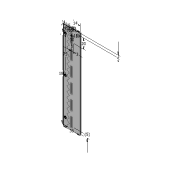
# Autodesk Inventor part: tray_side_top
Saved by Autodesk Inventor 2022 (Build 260153000, 153)
## iProperties
Created: 2022-05-19
Part Number: tray_side_top
Material: Generic
Document SubType Name: Modeling
Designer: Thomas
Density: 1 g/cm^3
Appearance: Default
Author: Thomas
Autodesk Inventor part; units mm, degrees
ref_plane "YZ Plane" through (0, 0, 0) normal (1, 0, 0) x (0, 1, 0)
ref_plane "XZ Plane" through (0, 0, 0) normal (0, 1, 0) x (-1, 0, 0)
ref_plane "XY Plane" through (0, 0, 0) normal (0, 0, 1) x (1, 0, 0)
sketch "Sketch1" plane through (0, 0, 0) normal (0, 0, 1) x (1, 0, 0)
  line L0 (0, 0) -> (-35, 0)
  line L1 (-35, 0) -> (-35, -180)
  line L2 (-35, -180) -> (0, -180)
  line L3 (0, -180) -> (0, 0)
  line L4 (-17, -5) -> (-14, -5)
  line L5 (-14, -5) -> (-14, -25)
  line L6 (-14, -25) -> (-17, -25)
  line L7 (-17, -25) -> (-17, -5)
  line L8 (-17, -35) -> (-14, -35)
  line L9 (-14, -35) -> (-14, -55)
  line L10 (-14, -55) -> (-17, -55)
  line L11 (-17, -55) -> (-17, -35)
  line L12 (-17, -65) -> (-14, -65)
  line L13 (-14, -65) -> (-14, -85)
  line L14 (-14, -85) -> (-17, -85)
  line L15 (-17, -85) -> (-17, -65)
  line L16 (-17, -95) -> (-14, -95)
  line L17 (-14, -95) -> (-14, -115)
  line L18 (-14, -115) -> (-17, -115)
  line L19 (-17, -115) -> (-17, -95)
  line L20 (-17, -125) -> (-14, -125)
  line L21 (-14, -125) -> (-14, -145)
  line L22 (-14, -145) -> (-17, -145)
  line L23 (-17, -145) -> (-17, -125)
  line L24 (-17, -155) -> (-14, -155)
  line L25 (-14, -155) -> (-14, -175)
  line L26 (-14, -175) -> (-17, -175)
  line L27 (-17, -175) -> (-17, -155)
  circle A0 centre (-31, -15) radius 2.075
  circle A1 centre (-31, -90) radius 2.075
  circle A2 centre (-31, -165) radius 2.075
  line L28 (-20, 0) -> (-25, -5)
  line L29 (-25, -5) -> (-20, -10)
  line L30 (-20, -10) -> (-25, -15)
  line L31 (-25, -15) -> (-20, -20)
  line L32 (-20, -20) -> (-25, -25)
  line L33 (-25, -25) -> (-20, -30)
  line L34 (-20, -30) -> (-25, -35)
  line L35 (-25, -35) -> (-20, -40)
  line L36 (-20, -40) -> (-25, -45)
  line L37 (-25, -45) -> (-20, -50)
  line L38 (-20, -50) -> (-25, -55)
  line L39 (-25, -55) -> (-20, -60)
  line L40 (-20, -60) -> (-25, -65)
  line L41 (-25, -65) -> (-20, -70)
  line L42 (-20, -70) -> (-25, -75)
  line L43 (-25, -75) -> (-20, -80)
  line L44 (-20, -80) -> (-25, -85)
  line L45 (-25, -85) -> (-20, -90)
  line L46 (-20, -90) -> (-25, -95)
  line L47 (-25, -95) -> (-20, -100)
  line L48 (-20, -100) -> (-25, -105)
  line L49 (-25, -105) -> (-20, -110)
  line L50 (-20, -110) -> (-25, -115)
  line L51 (-25, -115) -> (-20, -120)
  line L52 (-20, -120) -> (-25, -125)
  line L53 (-25, -125) -> (-20, -130)
  line L54 (-20, -130) -> (-25, -135)
  line L55 (-25, -135) -> (-20, -140)
  line L56 (-20, -140) -> (-25, -145)
  line L57 (-25, -145) -> (-20, -150)
  line L58 (-20, -150) -> (-25, -155)
  line L59 (-25, -155) -> (-20, -160)
  line L60 (-20, -160) -> (-25, -165)
  line L61 (-25, -165) -> (-20, -170)
  line L62 (-20, -170) -> (-25, -175)
  line L63 (-25, -175) -> (-20, -180)
  dimension "d0" = 35
  dimension "d1" = 180
  dimension "d2" = 3
  dimension "d3" = 20
  dimension "d4" = 5
  dimension "d5" = 14
  dimension "d8" = 30
  dimension "d13" = 5
  dimension "d14" = 4.15
  dimension "d15" = 4
  dimension "d16" = 10
  dimension "d19" = 75
  dimension "d24" = 5
  dimension "d25" = 45
  dimension "d26" = 7.0711
  dimension "d27" = 7.0711
  dimension "d28" = 20
  dimension "d31" = 10
  constraints: 128 end point, 4 parallel, 3 centre point, 3 perpendicular, 3 vertical, 2 horizontal, 1 collinear, 1 point on line, 128 other
  measures "d0" distance of L2.end L1.end
  measures "d1" distance of L1.end L0.end
  measures "d2" distance of L5.end L6.end
  measures "d3" distance of L4.end L5.end
  measures "d4" distance between parallel lines of L0 L4
  measures "d5" distance between parallel lines of L3 L5
  measures "d8" distance of L4.start L8.start
  measures "d13" distance from line of L2 L25.end
  measures "d14" diameter of A0
  measures "d15" distance from line of L1 A0.centre
  measures "d16" distance from line of L4 A0.centre
  measures "d19" distance of A0.centre A1.centre
  measures "d24" horizontal distance of L28.start L28.end
  measures "d25" angle of L28 L0
  measures "d26" distance of L28.start L28.end
  measures "d27" distance of L28.end L29.end
  measures "d28" distance from line of L3 L28.start
  measures "d31" distance of L28.start L30.start
extrude "Extrusion1" add sketch "Sketch1" against normal blind 2
extrude "Extrusion2" add sketch "Sketch1" along normal blind 2.5 contours L3 L2 L63 L62 L61 L60 L59 L58 L57 L56 L55 L54 L53 L52 L51 L50 L49 L48 L47 L46 L45 L44 L43 L42 L41 L40 L39 L38 L37 L36 L35 L34 L33 L32 L31 L30 L29 L28 L0
equation "\"d16\" = 0.5 * d3"
equation "\"d27\" = d26"
body "Solid1"
